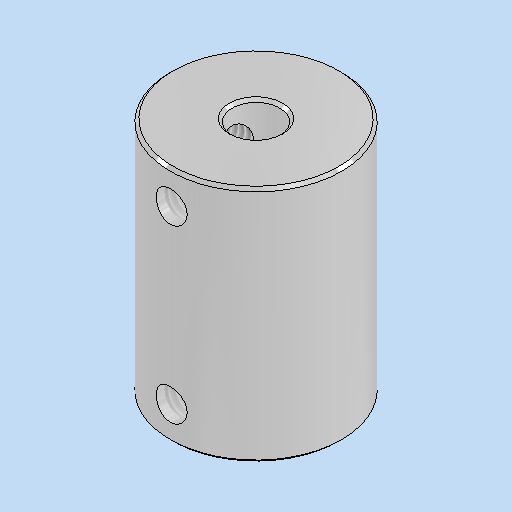
# Autodesk Inventor part: spring-shaft-coupler
Saved by Autodesk Inventor 2025 (Build 290162000, 162)
## iProperties
Created: 2025-06-05
Part Number: spring-shaft-coupler
Material: Aluminum 6061-AHC
Document SubType Name: Modeling
Designer: kuzmin
Density: 2.7 g/cm^3
Appearance: Aluminum - Dark
Author: kuzmin
Autodesk Inventor part; units mm, degrees
ref_plane "YZ Plane" through (0, 0, 0) normal (1, 0, 0) x (0, 1, 0)
ref_plane "XZ Plane" through (0, 0, 0) normal (0, 1, 0) x (-1, 0, 0)
ref_plane "XY Plane" through (0, 0, 0) normal (0, 0, 1) x (1, 0, 0)
sketch "Sketch1" plane through (0, 0, 0) normal (0, 0, 1) x (1, 0, 0)
  line L0 (0, -12.5) -> (0, 12.5)
  line L1 (9, 12.5) -> (9, -12.5)
  line L2 (9, -12.5) -> (4, -12.5)
  line L3 (4, -12.5) -> (4, 5.5)
  line L4 (4, 5.5) -> (2.5, 5.5)
  line L5 (2.5, 5.5) -> (2.5, 12.5)
  line L6 (2.5, 12.5) -> (9, 12.5)
  point P0 (0, 0)
  point P1 (0, 0)
  dimension "d0" = 18
  dimension "d1" = 25
  dimension "d2" = 8
  dimension "d3" = 5
  dimension "d4" = 18
  constraints: 14 end point, 3 perpendicular, 2 horizontal alignment, 1 coincident, 1 horizontal, 1 midpoint, 1 vertical
  measures "d0" diameter of L1 L0
  measures "d1" distance of L1.start L1.end
  measures "d2" diameter of L3 L0
  measures "d3" diameter of L5 L0
  measures "d4" distance of L2.end L3.end
revolve "Revolution1" add sketch "Sketch1" angle 360 about axis through (0, -12.5, 0) along (0, 1, 0)
sketch "Sketch2" plane through (0, 0, 0) normal (1, 0, 0) x (0, 1, 0)
  line L0 (12.5, -2.5) -> (12.5, 2.5) projected
  line L1 (-12.5, -4) -> (-12.5, 4) projected
  point P0 (0, 0)
  point P1 (9, 0)
  point P2 (-9, 0)
  dimension "d6" = 3.5
  dimension "d7" = 3.5
  constraints: 2 horizontal alignment
  measures "d6" distance from line of L0 point (9, 0)
  measures "d7" distance from line of L1 point (-9, 0)
hole "Hole1" at (0, 9, 0) at (0, -9, 0) direction (-1, 0, 0) diameter 3.242 end through all thread size "M4x0.7" class "6H" standard "ANSI Metric M Profile"
chamfer "Chamfer1" distance 0.3 angle 45 4 edges at (-9, 12.5, 0) (-2.5, 12.5, 0) (-9, -12.5, 0) (-4, -12.5, 0)
pattern_circular "Circular Pattern1" count 2 over 90 about axis through (0, 0, 0) along (0, 1, 0) of "Hole1"
body "Solid1"
